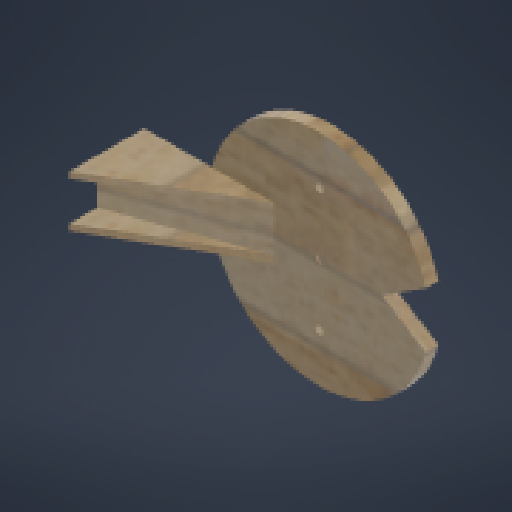
# Autodesk Inventor part: Base
Saved by Autodesk Inventor 2026.2 (Build 302298000, 298)
## iProperties
Created: 2026-03-02
Part Number: Base
Material: Wood (Maple)
Document SubType Name: Modeling
Designer: abdul
Density: 0.67 g/cm^3
Appearance: Natural Maple - Glossy Dark Tint
Author: abdul
Autodesk Inventor part; units mm, degrees
ref_plane "YZ Plane" through (0, 0, 0) normal (1, 0, 0) x (0, 1, 0)
sketch "Sketch1" plane through (0, 0, 0) normal (0, 0, 1) x (1, 0, 0)
  circle A0 centre (0, 0) radius 85
  line L0 (0, -85) -> (0, 85)
  line L1 (-85, 0) -> (85, 0)
  circle A1 centre (0, -47.5) radius 3.175
  circle A2 centre (0, 47.5) radius 3.175
  line L2 (82.2887, 21.2973) -> (48.4298, 0)
  line L3 (48.4298, 0) -> (82.2887, -21.2973)
  dimension "d0" = 170
  dimension "d21" = 6.35
  dimension "d22" = 47.5
  dimension "d49" = 40
  dimension "d50" = 40
  dimension "d51" = 32.17
  constraints: 8 end point, 4 point on circle, 3 centre point, 2 midpoint, 2 point on line, 1 coincident, 1 horizontal, 1 symmetric about line, 1 vertical, 1 other
  measures "d0" diameter of A0
  measures "d21" diameter of A1
  measures "d22" vertical distance of L1.end A1.centre
  measures "d49" distance of L2.start L2.end
  measures "d50" distance of L2.end L3.end
  measures "d51" angle of L1 L2
extrude "Extrusion1" add sketch "Sketch1" along normal blind 10
sketch "Sketch2" plane through (0, 0, 0) normal (0, 0, -1) x (-1, 0, 0)
  line L0 (-20, -25) -> (20, -25)
  line L1 (20, -25) -> (20, 25)
  line L2 (20, 25) -> (-20, 25)
  line L3 (-20, 25) -> (-20, -25)
  line L4 (0, -25) -> (0, 25)
  line L5 (5.3, -25) -> (5.3, 25)
  line L6 (-5.3, -25) -> (-5.3, 25)
  circle A0 centre (0, 0) radius 1.5
  point P0 (-5.3, -25)
  point P1 (5.3, -25)
  dimension "d3" = 40
  dimension "d4" = 50
  dimension "d18" = 3
  dimension "d25" = 5.3
  dimension "d27" = 10.6
  constraints: 14 end point, 6 parallel, 3 midpoint, 2 coincident, 2 perpendicular, 2 point on line, 1 centre point, 1 horizontal
  measures "d3" distance of L1.end L2.end
  measures "d4" distance of L0.end L1.end
  measures "d18" diameter of A0
  measures "d25" distance from line of point (0, 0) L5
  measures "d27" distance between parallel lines of L5 L6
extrude "Extrusion2" add sketch "Sketch2" along normal blind 3 contours L3 L2 L6 L0 | L5 L2 L1 L0
extrude "Extrusion3" add sketch "Sketch2" along normal blind 0.5 contours L6 L2 L4 A0 L0 | L4 A0 L2 L5 L0 | A0 L4 | L4 A0
extrude "Extrusion4" cut sketch "Sketch2" along normal through all both and the other way through all contours A0 L4 | L4 A0
extrude "Extrusion5" cut sketch "Sketch1" along normal through all contours A2 L0 | L0 A2 | A1 L0 | L0 A1
thread "Thread1" size "M3x0.5" class "6H" standard "ANSI Metric M Profile" length 77
sketch "Sketch3" plane through (0, 0, 10) normal (0, 0, 1) x (1, 0, 0)
  circle A0 centre (0, 0) radius 2.6
  dimension "d30" = 5.2
  constraints: 1 centre point, 1 coincident
  measures "d30" diameter of A0
extrude "Extrusion6" cut sketch "Sketch3" against normal blind 1.7
ref_plane "Work Plane1" through (0, 15, 0) normal (0, 1, 0) x (-1, 0, 0)
ref_plane "Work Plane2" through (0, -15, 0) normal (0, 1, 0) x (-1, 0, 0)
extrude "Extrusion9" cut sketch "Sketch1" along normal blind 10 contours L1 L2 A0 | A0 L3 L1
body "Solid1"
